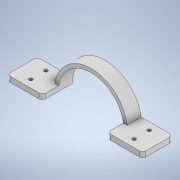
# Autodesk Inventor part: vydacha_2
Saved by Autodesk Inventor 2020 (Build 240168000, 168)
## iProperties
Created: 2022-07-26
Part Number: vydacha_2
Material: Типовые
Document SubType Name: Modeling
Designer: akapu
Density: 1 g/cm^3
Appearance: По умолчанию
Author: akapu
Autodesk Inventor part; units mm, degrees
ref_plane "YZ Plane" through (0, 0, 0) normal (1, 0, 0) x (0, 1, 0)
ref_plane "XZ Plane" through (0, 0, 0) normal (0, 1, 0) x (-1, 0, 0)
ref_plane "XY Plane" through (0, 0, 0) normal (0, 0, 1) x (1, 0, 0)
sketch "Эскиз1" plane through (0, 0, 0) normal (0, 0, 1) x (1, 0, 0)
  circle A0 centre (0, 0) radius 30.5
  circle A1 centre (0, 0) radius 34
  line L0 (0, 0) -> (-48.0635, 0)
  line L1 (-48.0635, 0) -> (48.0635, 0)
  line L2 (-48.0635, 0) -> (-63.0635, 0)
  line L3 (48.0635, 0) -> (63.0635, 0)
  line L4 (-63.0635, 0) -> (-63.0635, 5)
  line L5 (-63.0635, 5) -> (48.0635, 5)
  line L6 (48.0635, 5) -> (48.0635, 0)
  line L7 (63.0635, 0) -> (63.0635, 5)
  line L8 (63.0635, 5) -> (48.0635, 5)
  point P0 (-30.5, 0)
  point P1 (30.5, 0)
  point P2 (34, 0)
  point P3 (-34, 0)
  point P4 (33.6303, 5)
  point P5 (-33.6303, 5)
  dimension "d0" = 61
  dimension "d1" = 68
  dimension "d2" = 48.0635
  dimension "d3" = 96.127
  dimension "d4" = 15
  dimension "d5" = 15
  dimension "d9" = 5
  constraints: 18 end point, 3 perpendicular, 2 centre point, 2 coincident, 2 horizontal, 2 point on line, 2 vertical
  measures "d0" diameter of A0
  measures "d1" diameter of A1
  measures "d2" distance of L0.start L0.end
  measures "d3" distance of L0.end L1.end
  measures "d4" distance of L0.end L2.end
  measures "d5" distance of L1.end L3.end
  measures "d9" distance of L2.end L4.end
extrude "Выдавливание1" add sketch "Эскиз1" along normal blind 13 contours A0 L5 A1 L1 | A0 L5 A1 | L0 A1 L5 A0 | A1 L5 L6 L1 | L0 L2 L4 L5 A1 | L6 L8 L7 L3
sketch "Эскиз2" plane through (0, 0, 13) normal (0, 0, 1) x (1, 0, 0)
  circle A0 centre (0, 0) radius 30.5
  line L0 (-63.0635, 0) -> (-30.5, 0) projected
  line L1 (-63.0635, 0) -> (-30.0874, 0)
  line L2 (-30.0874, 0) -> (-30.0874, 5)
  line L3 (-30.0874, 5) -> (-63.0635, 5)
  line L4 (-63.0635, 5) -> (-63.0635, 0)
  line L5 (30.5, 0) -> (63.0635, 0) projected
  arc A1 (30.5, 0) -> (-30.5, 0) centre (0, 0) ccw projected
  line L6 (63.0635, 0) -> (30.0874, 0)
  line L7 (30.0874, 0) -> (30.0874, 5)
  line L8 (30.0874, 5) -> (63.0635, 5)
  line L9 (63.0635, 5) -> (63.0635, 0)
  constraints: 16 end point, 4 parallel, 2 horizontal, 2 perpendicular, 2 point on circle, 1 centre point, 1 coincident, 1 point on line
extrude "Выдавливание2" add sketch "Эскиз2" along normal blind 15 contours A0 L8 L9 L5 | L0 L4 L3 A0
sketch "Эскиз3" plane through (-63.0635, 5, 0) normal (0, 1, 0) x (1, 0, 0)
  line L0 (0, 0) -> (32.5635, 0) projected
  line L1 (0, 0) -> (15, 0)
  line L2 (15, 0) -> (15, -7)
  line L3 (15, -7) -> (15, -21)
  line L4 (93.5635, 0) -> (126.127, 0) projected
  line L5 (126.127, 0) -> (111.127, 0)
  line L6 (111.127, 0) -> (111.127, -7)
  line L7 (111.127, -7) -> (111.127, -21)
  circle A0 centre (111.127, -21) radius 1.6
  circle A1 centre (111.127, -7) radius 1.6
  circle A2 centre (15, -21) radius 1.6
  circle A3 centre (15, -7) radius 1.6
  point P0 (63.0635, 0)
  dimension "d12" = 15
  dimension "d13" = 7
  dimension "d14" = 14
  dimension "d15" = 15
  dimension "d16" = 3.2
  dimension "d17" = 3.2
  dimension "d18" = 3.2
  dimension "d19" = 3.2
  constraints: 12 end point, 4 centre point, 4 coincident, 4 point on line, 2 perpendicular
  measures "d12" distance of L0.start L1.end
  measures "d13" distance of L1.end L2.end
  measures "d14" distance of L2.end L3.end
  measures "d15" distance of L4.end L5.end
  measures "d16" diameter of A0
  measures "d17" diameter of A1
  measures "d18" diameter of A2
  measures "d19" diameter of A3
extrude "Выдавливание3" cut sketch "Эскиз3" against normal blind 15
fillet "Сопряжение1" radius 3 6 edges at (30.3967, 2.5085, 28) (63.0635, 2.5, 28) (63.0635, 2.5, 0) (-63.0635, 2.5, 0) (-63.0635, 2.5, 28) (-30.3967, 2.5085, 28)
